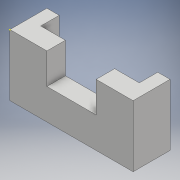
# Autodesk Inventor part: P3-5
Saved by Autodesk Inventor 2017 (Build 210142000, 142)
## iProperties
Created: 2017-02-12
Part Number: P3-5
Material: Generic
Document SubType Name: Modeling
Designer: Schaffel
Density: 1 g/cm^3
Appearance: Default
Author: Schaffel
Autodesk Inventor part; units mm, degrees
ref_plane "YZ Plane" through (0, 0, 0) normal (1, 0, 0) x (0, 1, 0)
ref_plane "XZ Plane" through (0, 0, 0) normal (0, 1, 0) x (-1, 0, 0)
ref_plane "XY Plane" through (0, 0, 0) normal (0, 0, 1) x (1, 0, 0)
sketch "Sketch1" plane through (0, 0, 0) normal (0, 1, 0) x (-1, 0, 0)
  point P0 (0, 0)
sketch "Sketch2" plane through (0, 0, 0) normal (0, 1, 0) x (-1, 0, 0)
  line L0 (0, 0) -> (-30, 0)
  line L1 (-30, 0) -> (-30, -25)
  line L2 (-30, -25) -> (-70, -25)
  line L3 (-70, -25) -> (-70, 0)
  line L4 (-70, 0) -> (-100, 0)
  line L5 (-100, 0) -> (-100, -50)
  line L6 (-100, -50) -> (0, -50)
  line L7 (0, -50) -> (0, 0)
  dimension "d0" = 30
  dimension "d1" = 25
  dimension "d2" = 40
  constraints: 16 end point, 6 perpendicular, 2 point on line, 1 horizontal
  measures "d0" distance of L0.start L0.end
  measures "d1" distance of L0.end L1.end
  measures "d2" distance of L1.end L2.end
extrude "Extrusion1" add sketch "Sketch2" along normal blind 15
sketch "Sketch3" plane through (0, 15, 0) normal (0, 1, 0) x (1, 0, 0)
  line L0 (0, 0) -> (10, 0)
  line L1 (0, 0) -> (30, 0) projected
  line L2 (10, 40) -> (10, 0)
  line L3 (10, 40) -> (40, 40)
  line L4 (40, 40) -> (40, 50)
  line L5 (0, 50) -> (0, 0) projected
  line L6 (40, 50) -> (0, 50)
  line L7 (0, 50) -> (0, 0)
  line L8 (100, 0) -> (100, 50) projected
  line L9 (100, 0) -> (100, 50)
  line L10 (100, 50) -> (60, 50)
  line L11 (100, 50) -> (0, 50) projected
  line L12 (60, 40) -> (60, 50)
  line L13 (60, 40) -> (90, 40)
  line L14 (90, 40) -> (90, 0)
  line L15 (70, 0) -> (100, 0) projected
  line L16 (100, 0) -> (90, 0)
  constraints: 24 end point, 6 perpendicular, 3 point on line, 2 collinear, 2 horizontal
extrude "Extrusion2" add sketch "Sketch3" along normal blind 15
body "Solid1"
